Autodesk Fusion 360 part; units mm, degrees
(part 4 of 4)
  circle A338 centre (0, 0) radius 300
  spline S338 degree 3 poles (61.4407, -278.2986) (59.9759, -276.2105) (58.7077, -274.2475) (57.6132, -272.4294) knots 0 0 0 0 1 1 1 1
  spline S339 degree 3 poles (278.2308, -11.1655) (280.2066, -11.94) (282.3543, -12.8615) (284.6582, -13.9559) knots 0 0 0 0 1 1 1 1
  spline S340 degree 3 poles (276.3178, -10.4408) (276.936, -10.6668) (277.5738, -10.908) (278.2308, -11.1655) knots 0 0 0 0 1 1 1 1
  arc A339 (282.974, -33.9233) -> (283.4279, -29.8949) centre (0, 0) ccw
  spline S341 degree 3 poles (276.1699, -35.5976) (275.4792, -35.7415) (274.81, -35.8724) (274.1626, -35.9916) knots 0 0 0 0 1 1 1 1
  spline S342 degree 3 poles (275.2312, -42.2473) (277.1078, -43.2382) (279.1389, -44.3943) (281.3058, -45.7398) knots 0 0 0 0 1 1 1 1
  arc A340 (276.0555, -10.0506) -> (276.3178, -10.4408) centre (276.4552, -10.0652) ccw
  arc A341 (276.0555, -10.0506) -> (276.1847, -5.4437) centre (0, 0) ccw
  arc A342 (71.6656, -267.0666) -> (71.2268, -266.8977) centre (71.3299, -267.2842) ccw
  spline S343 degree 3 poles (280.6267, -49.7364) (278.137, -50.2907) (275.8381, -50.7111) (273.7395, -51.0266) knots 0 0 0 0 1 1 1 1
  arc A343 (280.6267, -49.7364) -> (281.3058, -45.7398) centre (0, 0) ccw
  arc A344 (273.1944, -40.8958) -> (273.4114, -41.313) centre (273.59, -40.9551) ccw
  spline S344 degree 3 poles (272.4294, -57.6132) (274.2475, -58.7077) (276.2105, -59.9759) (278.2986, -61.4407) knots 0 0 0 0 1 1 1 1
  spline S345 degree 3 poles (277.3965, -65.393) (274.8797, -65.8068) (272.5608, -66.0977) (270.4478, -66.295) knots 0 0 0 0 1 1 1 1
  arc A345 (257.2447, -100.662) -> (257.3634, -101.1169) centre (257.6171, -100.8077) ccw
  arc A346 (236.7485, -142.3298) -> (239.0901, -138.3603) centre (0, 0) ccw
  arc A347 (262.5234, -110.9347) -> (264.0748, -107.1894) centre (0, 0) ccw
  spline S346 degree 3 poles (252.7789, -116.7899) (254.3079, -118.2616) (255.9395, -119.9348) (257.6492, -121.8275) knots 0 0 0 0 1 1 1 1
  arc A348 (246.8902, -124.5221) -> (246.4719, -124.7367) centre (246.8288, -124.9173) ccw
  arc A349 (240.232, -153.3416) -> (242.3888, -149.9091) centre (0, 0) ccw
  arc A350 (244.3566, -128.8313) -> (244.4236, -129.2967) centre (244.7104, -129.0178) ccw
  arc A351 (236.7485, -142.3298) -> (236.7894, -142.7982) centre (237.0914, -142.5359) ccw
  spline S347 degree 3 poles (255.5218, -110.66) (254.8182, -110.607) (254.1389, -110.5476) (253.4839, -110.4829) knots 0 0 0 0 1 1 1 1
  arc A352 (248.452, -139.6305) -> (250.4129, -136.0824) centre (0, 0) ccw
  spline S348 degree 3 poles (248.9151, -124.8131) (248.2155, -124.7208) (247.5406, -124.6234) (246.8902, -124.5221) knots 0 0 0 0 1 1 1 1
  spline S349 degree 3 poles (248.452, -139.6305) (245.919, -139.3314) (243.6102, -138.969) (241.5251, -138.5736) knots 0 0 0 0 1 1 1 1
  arc A353 (262.4841, -86.0798) -> (263.8837, -81.6887) centre (0, 0) ccw
  arc A354 (262.4841, -86.0798) -> (262.6282, -86.5274) centre (262.8642, -86.2044) ccw
  spline S350 degree 3 poles (238.1131, -144.3578) (239.4677, -145.9914) (240.9017, -147.8368) (242.3888, -149.9091) knots 0 0 0 0 1 1 1 1
  spline S351 degree 3 poles (229.6443, -157.4818) (230.9052, -159.1888) (232.2335, -161.1117) (233.602, -163.2641) knots 0 0 0 0 1 1 1 1
  arc A355 (231.3958, -151.382) -> (230.9561, -151.5485) centre (231.2905, -151.7679) ccw
  spline S352 degree 3 poles (258.9296, -102.4328) (260.5388, -103.8164) (262.2616, -105.3955) (264.0748, -107.1894) knots 0 0 0 0 1 1 1 1
  spline S353 degree 3 poles (251.2888, -115.3883) (251.7735, -115.8336) (252.2705, -116.3006) (252.7789, -116.7899) knots 0 0 0 0 1 1 1 1
  arc A356 (257.2447, -100.662) -> (258.8882, -96.3563) centre (0, 0) ccw
  spline S354 degree 3 poles (266.3051, -81.3548) (265.6, -81.381) (264.9183, -81.398) (264.2602, -81.407) knots 0 0 0 0 1 1 1 1
  arc A357 (251.1958, -114.9274) -> (251.2888, -115.3883) centre (251.5595, -115.0938) ccw
  spline S355 degree 3 poles (262.6282, -86.5274) (263.1597, -86.9156) (263.7058, -87.324) (264.2658, -87.7533) knots 0 0 0 0 1 1 1 1
  arc A358 (259.2799, -96.0962) -> (258.8882, -96.3563) centre (259.2631, -96.4958) ccw
  spline S356 degree 3 poles (262.5234, -110.9347) (259.9728, -110.9211) (257.638, -110.8195) (255.5218, -110.66) knots 0 0 0 0 1 1 1 1
  arc A359 (244.3566, -128.8313) -> (246.4719, -124.7367) centre (0, 0) ccw
  arc A360 (255.8902, -125.48) -> (257.6492, -121.8275) centre (0, 0) ccw
  spline S357 degree 3 poles (255.8902, -125.48) (253.3445, -125.3234) (251.019, -125.091) (248.9151, -124.8131) knots 0 0 0 0 1 1 1 1
  spline S358 degree 3 poles (244.4236, -129.2967) (244.8826, -129.7685) (245.3526, -130.2625) (245.8327, -130.7796) knots 0 0 0 0 1 1 1 1
  spline S359 degree 3 poles (233.3753, -151.898) (232.6905, -151.7279) (232.0307, -151.5555) (231.3958, -151.382) knots 0 0 0 0 1 1 1 1
  spline S360 degree 3 poles (236.7894, -142.7982) (237.2212, -143.295) (237.6627, -143.8146) (238.1131, -144.3578) knots 0 0 0 0 1 1 1 1
  arc A361 (273.2935, -80.8439) -> (274.4157, -76.9484) centre (0, 0) ccw
  spline S361 degree 3 poles (240.232, -153.3416) (237.7197, -152.901) (235.4349, -152.4097) (233.3753, -151.898) knots 0 0 0 0 1 1 1 1
  arc A362 (264.2602, -81.407) -> (263.8837, -81.6887) centre (264.2658, -81.807) ccw
  spline S362 degree 3 poles (228.4101, -155.8505) (228.8134, -156.3707) (229.2251, -156.9142) (229.6443, -157.4818) knots 0 0 0 0 1 1 1 1
  arc A363 (228.3956, -155.3805) -> (228.4101, -155.8505) centre (228.7263, -155.6055) ccw
  spline S363 degree 3 poles (268.3306, -96.0404) (265.7832, -96.1698) (263.4464, -96.1992) (261.3246, -96.1587) knots 0 0 0 0 1 1 1 1
  arc A364 (231.2561, -166.5703) -> (233.602, -163.2641) centre (0, 0) ccw
  arc A365 (251.1958, -114.9274) -> (253.0782, -110.7207) centre (0, 0) ccw
  spline S364 degree 3 poles (241.5251, -138.5736) (240.8319, -138.4421) (240.1635, -138.307) (239.5198, -138.1694) knots 0 0 0 0 1 1 1 1
  spline S365 degree 3 poles (273.2935, -80.8439) (270.7574, -81.1159) (268.4259, -81.2764) (266.3051, -81.3548) knots 0 0 0 0 1 1 1 1
  spline S366 degree 3 poles (245.8327, -130.7796) (247.2768, -132.3347) (248.812, -134.0968) (250.4129, -136.0824) knots 0 0 0 0 1 1 1 1
  arc A366 (228.3956, -155.3805) -> (230.9561, -151.5485) centre (0, 0) ccw
  spline S367 degree 3 poles (261.3246, -96.1587) (260.6191, -96.1452) (259.9375, -96.124) (259.2799, -96.0962) knots 0 0 0 0 1 1 1 1
  spline S368 degree 3 poles (231.2561, -166.5703) (228.7725, -165.9895) (226.5188, -165.3708) (224.4912, -164.7445) knots 0 0 0 0 1 1 1 1
  spline S369 degree 3 poles (220.453, -170.1103) (221.6162, -171.8853) (222.8345, -173.8797) (224.0802, -176.1054) knots 0 0 0 0 1 1 1 1
  spline S370 degree 3 poles (224.4912, -164.7445) (223.817, -164.5362) (223.1679, -164.3272) (222.5437, -164.1184) knots 0 0 0 0 1 1 1 1
  arc A367 (219.324, -167.9423) -> (222.0953, -164.2599) centre (0, 0) ccw
  arc A368 (239.5198, -138.1694) -> (239.0901, -138.3603) centre (239.4363, -138.5606) ccw
  arc A369 (222.5437, -164.1184) -> (222.0953, -164.2599) centre (222.4169, -164.4977) ccw
  spline S371 degree 3 poles (219.3122, -168.4123) (219.6856, -168.9543) (220.0662, -169.5201) (220.453, -170.1103) knots 0 0 0 0 1 1 1 1
  spline S372 degree 3 poles (264.2658, -87.7533) (265.9499, -89.0445) (267.7586, -90.5246) (269.6695, -92.214) knots 0 0 0 0 1 1 1 1
  arc A370 (253.4839, -110.4829) -> (253.0782, -110.7207) centre (253.4447, -110.881) ccw
  arc A371 (268.3306, -96.0404) -> (269.6695, -92.214) centre (0, 0) ccw
  spline S373 degree 3 poles (257.3634, -101.1169) (257.8723, -101.5344) (258.3946, -101.9727) (258.9296, -102.4328) knots 0 0 0 0 1 1 1 1
  spline S374 degree 3 poles (200.0205, -193.7236) (200.9776, -195.6177) (201.965, -197.7359) (202.9537, -200.0871) knots 0 0 0 0 1 1 1 1
  spline S375 degree 3 poles (188.0034, -202.769) (188.2808, -203.3659) (188.5612, -203.9875) (188.8436, -204.6341) knots 0 0 0 0 1 1 1 1
  arc A372 (188.0938, -202.3076) -> (191.4428, -199.1414) centre (0, 0) ccw
  arc A373 (176.4544, -212.5358) -> (176.3383, -212.9914) centre (176.71, -212.8436) ccw
  arc A374 (212.9914, -176.3383) -> (212.5358, -176.4544) centre (212.8436, -176.71) ccw
  spline S376 degree 3 poles (200.0871, -202.9537) (197.7359, -201.965) (195.6177, -200.9776) (193.7236, -200.0205) knots 0 0 0 0 1 1 1 1
  spline S377 degree 3 poles (188.3926, -213.8534) (186.1006, -212.7344) (184.041, -211.6298) (182.2036, -210.568) knots 0 0 0 0 1 1 1 1
  spline S378 degree 3 poles (188.8436, -204.6341) (189.6931, -206.5789) (190.5602, -208.7491) (191.4154, -211.152) knots 0 0 0 0 1 1 1 1
  spline S379 degree 3 poles (177.0726, -214.9007) (177.8117, -216.89) (178.5557, -219.1055) (179.2749, -221.5526) knots 0 0 0 0 1 1 1 1
  spline S380 degree 3 poles (210.568, -182.2036) (211.6298, -184.041) (212.7344, -186.1006) (213.8534, -188.3926) knots 0 0 0 0 1 1 1 1
  arc A375 (155.8505, -228.4101) -> (155.3805, -228.3956) centre (155.6055, -228.7263) ccw
  spline S381 degree 3 poles (157.4818, -229.6443) (156.9142, -229.2251) (156.3707, -228.8134) (155.8505, -228.4101) knots 0 0 0 0 1 1 1 1
  arc A376 (199.1414, -191.4428) -> (202.3076, -188.0938) centre (0, 0) ccw
  arc A377 (149.9091, -242.3888) -> (153.3416, -240.232) centre (0, 0) ccw
  arc A378 (151.5485, -230.9561) -> (151.382, -231.3958) centre (151.7679, -231.2905) ccw
  spline S382 degree 3 poles (214.9007, -177.0726) (214.2393, -176.8269) (213.6029, -176.5818) (212.9914, -176.3383) knots 0 0 0 0 1 1 1 1
  arc A379 (200.0871, -202.9537) -> (202.9537, -200.0871) centre (0, 0) ccw
  spline S383 degree 3 poles (193.7236, -200.0205) (193.0938, -199.7023) (192.489, -199.3874) (191.9086, -199.077) knots 0 0 0 0 1 1 1 1
  arc A380 (151.5485, -230.9561) -> (155.3805, -228.3956) centre (0, 0) ccw
  arc A381 (202.769, -188.0034) -> (202.3076, -188.0938) centre (202.6005, -188.3662) ccw
  spline S384 degree 3 poles (211.152, -191.4154) (208.7491, -190.5602) (206.5789, -189.6931) (204.6341, -188.8436) knots 0 0 0 0 1 1 1 1
  spline S385 degree 3 poles (204.6341, -188.8436) (203.9875, -188.5612) (203.3659, -188.2808) (202.769, -188.0034) knots 0 0 0 0 1 1 1 1
  arc A382 (191.9086, -199.077) -> (191.4428, -199.1414) centre (191.72, -199.4298) ccw
  arc A383 (219.324, -167.9423) -> (219.3122, -168.4123) centre (219.6416, -168.1855) ccw
  spline S386 degree 3 poles (176.1054, -224.0802) (173.8797, -222.8345) (171.8853, -221.6162) (170.1103, -220.453) knots 0 0 0 0 1 1 1 1
  arc A384 (176.1054, -224.0802) -> (179.2749, -221.5526) centre (0, 0) ccw
  arc A385 (163.2641, -233.602) -> (166.5703, -231.2561) centre (0, 0) ccw
  spline S387 degree 3 poles (164.7445, -224.4912) (165.3708, -226.5188) (165.9895, -228.7725) (166.5703, -231.2561) knots 0 0 0 0 1 1 1 1
  arc A386 (168.4123, -219.3122) -> (167.9423, -219.324) centre (168.1855, -219.6416) ccw
  arc A387 (188.0938, -202.3076) -> (188.0034, -202.769) centre (188.3662, -202.6005) ccw
  arc A388 (211.152, -191.4154) -> (213.8534, -188.3926) centre (0, 0) ccw
  spline S388 degree 3 poles (182.2036, -210.568) (181.5927, -210.2149) (181.0064, -209.8667) (180.4443, -209.5242) knots 0 0 0 0 1 1 1 1
  arc A389 (209.5624, -179.9757) -> (209.5242, -180.4443) centre (209.8658, -180.2363) ccw
  arc A390 (176.4544, -212.5358) -> (179.9757, -209.5624) centre (0, 0) ccw
  spline S389 degree 3 poles (199.077, -191.9086) (199.3874, -192.489) (199.7023, -193.0938) (200.0205, -193.7236) knots 0 0 0 0 1 1 1 1
  arc A391 (180.4443, -209.5242) -> (179.9757, -209.5624) centre (180.2363, -209.8658) ccw
  arc A392 (164.2599, -222.0953) -> (164.1184, -222.5437) centre (164.4977, -222.4169) ccw
  spline S390 degree 3 poles (164.1184, -222.5437) (164.3272, -223.1679) (164.5362, -223.817) (164.7445, -224.4912) knots 0 0 0 0 1 1 1 1
  arc A393 (209.5624, -179.9757) -> (212.5358, -176.4544) centre (0, 0) ccw
  spline S391 degree 3 poles (170.1103, -220.453) (169.5201, -220.0662) (168.9543, -219.6856) (168.4123, -219.3122) knots 0 0 0 0 1 1 1 1
  arc A394 (164.2599, -222.0953) -> (167.9423, -219.324) centre (0, 0) ccw
  spline S392 degree 3 poles (163.2641, -233.602) (161.1117, -232.2335) (159.1888, -230.9052) (157.4818, -229.6443) knots 0 0 0 0 1 1 1 1
  spline S393 degree 3 poles (151.898, -233.3753) (152.4097, -235.4349) (152.901, -237.7197) (153.3416, -240.232) knots 0 0 0 0 1 1 1 1
  arc A395 (188.3926, -213.8534) -> (191.4154, -211.152) centre (0, 0) ccw
  spline S394 degree 3 poles (151.382, -231.3958) (151.5555, -232.0307) (151.7279, -232.6905) (151.898, -233.3753) knots 0 0 0 0 1 1 1 1
  spline S395 degree 3 poles (176.3383, -212.9914) (176.5818, -213.6029) (176.8269, -214.2393) (177.0726, -214.9007) knots 0 0 0 0 1 1 1 1
  arc A396 (221.5526, -179.2749) -> (224.0802, -176.1054) centre (0, 0) ccw
  spline S396 degree 3 poles (209.5242, -180.4443) (209.8667, -181.0064) (210.2149, -181.5927) (210.568, -182.2036) knots 0 0 0 0 1 1 1 1
  spline S397 degree 3 poles (221.5526, -179.2749) (219.1055, -178.5557) (216.89, -177.8117) (214.9007, -177.0726) knots 0 0 0 0 1 1 1 1
  arc A397 (199.1414, -191.4428) -> (199.077, -191.9086) centre (199.4298, -191.72) ccw
  spline S398 degree 3 poles (166.5703, 231.2561) (165.9895, 228.7725) (165.3708, 226.5188) (164.7445, 224.4912) knots 0 0 0 0 1 1 1 1
  arc A398 (167.9423, 219.324) -> (164.2599, 222.0953) centre (0, 0) ccw
  spline S399 degree 3 poles (277.167, 26.7485) (276.5255, 26.4545) (275.9023, 26.1779) (275.2977, 25.9177) knots 0 0 0 0 1 1 1 1
  spline S400 degree 3 poles (155.8505, 228.4101) (156.3707, 228.8134) (156.9142, 229.2251) (157.4818, 229.6443) knots 0 0 0 0 1 1 1 1
  arc A399 (138.1694, 239.5198) -> (138.3603, 239.0901) centre (138.5606, 239.4363) ccw
  spline S401 degree 3 poles (168.4123, 219.3122) (168.9543, 219.6856) (169.5201, 220.0662) (170.1103, 220.453) knots 0 0 0 0 1 1 1 1
  spline S402 degree 3 poles (179.2749, 221.5526) (178.5557, 219.1055) (177.8117, 216.89) (177.0726, 214.9007) knots 0 0 0 0 1 1 1 1
  spline S403 degree 3 poles (276.1699, 35.5976) (278.2476, 35.165) (280.5193, 34.6163) (282.974, 33.9233) knots 0 0 0 0 1 1 1 1
  arc A400 (276.1847, 5.4437) -> (276.4685, 5.0688) centre (276.5847, 5.4516) ccw
  arc A401 (166.5703, 231.2561) -> (163.2641, 233.602) centre (0, 0) ccw
  spline S404 degree 3 poles (275.2312, 42.2473) (274.6072, 41.9178) (274.0004, 41.6067) (273.4114, 41.313) knots 0 0 0 0 1 1 1 1
  spline S405 degree 3 poles (170.1103, 220.453) (171.8853, 221.6162) (173.8797, 222.8345) (176.1054, 224.0802) knots 0 0 0 0 1 1 1 1
  arc A402 (275.2977, 25.9177) -> (275.0576, 25.5134) centre (275.4559, 25.5503) ccw
  spline S406 degree 3 poles (180.4443, 209.5242) (181.0064, 209.8667) (181.5927, 210.2149) (182.2036, 210.568) knots 0 0 0 0 1 1 1 1
  spline S407 degree 3 poles (139.6305, 248.452) (139.3314, 245.919) (138.969, 243.6102) (138.5736, 241.5251) knots 0 0 0 0 1 1 1 1
  arc A403 (179.9757, 209.5624) -> (176.4544, 212.5358) centre (0, 0) ccw
  spline S408 degree 3 poles (283.4279, 29.8949) (281.1889, 28.673) (279.0963, 27.6326) (277.167, 26.7485) knots 0 0 0 0 1 1 1 1
  arc A404 (275.445, 20.921) -> (275.0576, 25.5134) centre (0, 0) ccw
  spline S409 degree 3 poles (284.6582, 13.9559) (282.3543, 12.8615) (280.2066, 11.94) (278.2308, 11.1655) knots 0 0 0 0 1 1 1 1
  spline S410 degree 3 poles (144.3578, 238.1131) (145.9914, 239.4677) (147.8368, 240.9017) (149.9091, 242.3888) knots 0 0 0 0 1 1 1 1
  arc A405 (283.4279, 29.8949) -> (282.974, 33.9233) centre (0, 0) ccw
  arc A406 (155.3805, 228.3956) -> (155.8505, 228.4101) centre (155.6055, 228.7263) ccw
  spline S411 degree 3 poles (275.7494, 20.5626) (276.389, 20.4073) (277.0498, 20.239) (277.7315, 20.0566) knots 0 0 0 0 1 1 1 1
  spline S412 degree 3 poles (278.2308, 11.1655) (277.5738, 10.908) (276.936, 10.6668) (276.3178, 10.4408) knots 0 0 0 0 1 1 1 1
  arc A407 (273.8386, 36.3324) -> (273.1944, 40.8958) centre (0, 0) ccw
  spline S413 degree 3 poles (138.5736, 241.5251) (138.4421, 240.8319) (138.307, 240.1635) (138.1694, 239.5198) knots 0 0 0 0 1 1 1 1
  arc A408 (155.3805, 228.3956) -> (151.5485, 230.9561) centre (0, 0) ccw
  arc A409 (151.382, 231.3958) -> (151.5485, 230.9561) centre (151.7679, 231.2905) ccw
  arc A410 (179.9757, 209.5624) -> (180.4443, 209.5242) centre (180.2363, 209.8658) ccw
  arc A411 (281.3058, 45.7398) -> (280.6267, 49.7364) centre (0, 0) ccw
  spline S414 degree 3 poles (281.3058, 45.7398) (279.1389, 44.3943) (277.1078, 43.2382) (275.2312, 42.2473) knots 0 0 0 0 1 1 1 1
  arc A412 (179.2749, 221.5526) -> (176.1054, 224.0802) centre (0, 0) ccw
  arc A413 (176.3383, 212.9914) -> (176.4544, 212.5358) centre (176.71, 212.8436) ccw
  spline S415 degree 3 poles (177.0726, 214.9007) (176.8269, 214.2393) (176.5818, 213.6029) (176.3383, 212.9914) knots 0 0 0 0 1 1 1 1
  arc A414 (191.4154, 211.152) -> (188.3926, 213.8534) centre (0, 0) ccw
  arc A415 (273.8386, 36.3324) -> (274.1626, 35.9916) centre (274.2352, 36.385) ccw
  spline S416 degree 3 poles (277.7315, 20.0566) (279.7816, 19.5082) (282.0189, 18.833) (284.4309, 18.0035) knots 0 0 0 0 1 1 1 1
  arc A416 (276.1847, 5.4437) -> (276.0555, 10.0506) centre (0, 0) ccw
  spline S417 degree 3 poles (153.3416, 240.232) (152.901, 237.7197) (152.4097, 235.4349) (151.898, 233.3753) knots 0 0 0 0 1 1 1 1
  spline S418 degree 3 poles (151.898, 233.3753) (151.7279, 232.6905) (151.5555, 232.0307) (151.382, 231.3958) knots 0 0 0 0 1 1 1 1
  arc A417 (273.4114, 41.313) -> (273.1944, 40.8958) centre (273.59, 40.9551) ccw
  arc A418 (164.1184, 222.5437) -> (164.2599, 222.0953) centre (164.4977, 222.4169) ccw
  arc A419 (167.9423, 219.324) -> (168.4123, 219.3122) centre (168.1855, 219.6416) ccw
  spline S419 degree 3 poles (164.7445, 224.4912) (164.5362, 223.817) (164.3272, 223.1679) (164.1184, 222.5437) knots 0 0 0 0 1 1 1 1
  spline S420 degree 3 poles (273.7395, 51.0266) (275.8381, 50.7111) (278.137, 50.2907) (280.6267, 49.7364) knots 0 0 0 0 1 1 1 1
  arc A420 (284.6582, 13.9559) -> (284.4309, 18.0035) centre (0, 0) ccw
  arc A421 (142.3298, 236.7485) -> (142.7982, 236.7894) centre (142.5359, 237.0914) ccw
  spline S421 degree 3 poles (142.7982, 236.7894) (143.295, 237.2212) (143.8146, 237.6627) (144.3578, 238.1131) knots 0 0 0 0 1 1 1 1
  arc A422 (153.3416, 240.232) -> (149.9091, 242.3888) centre (0, 0) ccw
  spline S422 degree 3 poles (274.1626, 35.9916) (274.81, 35.8724) (275.4792, 35.7415) (276.1699, 35.5976) knots 0 0 0 0 1 1 1 1
  arc A423 (275.445, 20.921) -> (275.7494, 20.5626) centre (275.8439, 20.9513) ccw
  arc A424 (276.3178, 10.4408) -> (276.0555, 10.0506) centre (276.4552, 10.0652) ccw
  arc A425 (142.3298, 236.7485) -> (138.3603, 239.0901) centre (0, 0) ccw
  spline S423 degree 3 poles (157.4818, 229.6443) (159.1888, 230.9052) (161.1117, 232.2335) (163.2641, 233.602) knots 0 0 0 0 1 1 1 1
  arc A426 (213.8534, 188.3926) -> (211.152, 191.4154) centre (0, 0) ccw
  arc A427 (202.3076, 188.0938) -> (202.769, 188.0034) centre (202.6005, 188.3662) ccw
  spline S424 degree 3 poles (202.9537, 200.0871) (201.965, 197.7359) (200.9776, 195.6177) (200.0205, 193.7236) knots 0 0 0 0 1 1 1 1
  spline S425 degree 3 poles (188.8436, 204.6341) (188.5612, 203.9875) (188.2808, 203.3659) (188.0034, 202.769) knots 0 0 0 0 1 1 1 1
  spline S426 degree 3 poles (204.6341, 188.8436) (206.5789, 189.6931) (208.7491, 190.5602) (211.152, 191.4154) knots 0 0 0 0 1 1 1 1
  arc A428 (224.0802, 176.1054) -> (221.5526, 179.2749) centre (0, 0) ccw
  arc A429 (212.5358, 176.4544) -> (209.5624, 179.9757) centre (0, 0) ccw
  arc A430 (191.4428, 199.1414) -> (191.9086, 199.077) centre (191.72, 199.4298) ccw
  spline S427 degree 3 poles (224.0802, 176.1054) (222.8345, 173.8797) (221.6162, 171.8853) (220.453, 170.1103) knots 0 0 0 0 1 1 1 1
  spline S428 degree 3 poles (224.4912, 164.7445) (226.5188, 165.3708) (228.7725, 165.9895) (231.2561, 166.5703) knots 0 0 0 0 1 1 1 1
  spline S429 degree 3 poles (233.602, 163.2641) (232.2335, 161.1117) (230.9052, 159.1888) (229.6443, 157.4818) knots 0 0 0 0 1 1 1 1
  spline S430 degree 3 poles (229.6443, 157.4818) (229.2251, 156.9142) (228.8134, 156.3707) (228.4101, 155.8505) knots 0 0 0 0 1 1 1 1
  arc A431 (230.9561, 151.5485) -> (231.3958, 151.382) centre (231.2905, 151.7679) ccw
  spline S431 degree 3 poles (233.3753, 151.898) (235.4349, 152.4097) (237.7197, 152.901) (240.232, 153.3416) knots 0 0 0 0 1 1 1 1
  spline S432 degree 3 poles (231.3958, 151.382) (232.0307, 151.5555) (232.6905, 151.7279) (233.3753, 151.898) knots 0 0 0 0 1 1 1 1
  arc A432 (222.0953, 164.2599) -> (219.324, 167.9423) centre (0, 0) ccw
  arc A433 (202.9537, 200.0871) -> (200.0871, 202.9537) centre (0, 0) ccw
  spline S433 degree 3 poles (213.8534, 188.3926) (212.7344, 186.1006) (211.6298, 184.041) (210.568, 182.2036) knots 0 0 0 0 1 1 1 1
  spline S434 degree 3 poles (212.9914, 176.3383) (213.6029, 176.5818) (214.2393, 176.8269) (214.9007, 177.0726) knots 0 0 0 0 1 1 1 1
  spline S435 degree 3 poles (222.5437, 164.1184) (223.1679, 164.3272) (223.817, 164.5362) (224.4912, 164.7445) knots 0 0 0 0 1 1 1 1
  arc A434 (233.602, 163.2641) -> (231.2561, 166.5703) centre (0, 0) ccw
  arc A435 (242.3888, 149.9091) -> (240.232, 153.3416) centre (0, 0) ccw
  arc A436 (188.0034, 202.769) -> (188.0938, 202.3076) centre (188.3662, 202.6005) ccw
  arc A437 (230.9561, 151.5485) -> (228.3956, 155.3805) centre (0, 0) ccw
  spline S436 degree 3 poles (191.9086, 199.077) (192.489, 199.3874) (193.0938, 199.7023) (193.7236, 200.0205) knots 0 0 0 0 1 1 1 1
  spline S437 degree 3 poles (193.7236, 200.0205) (195.6177, 200.9776) (197.7359, 201.965) (200.0871, 202.9537) knots 0 0 0 0 1 1 1 1
  spline S438 degree 3 poles (210.568, 182.2036) (210.2149, 181.5927) (209.8667, 181.0064) (209.5242, 180.4443) knots 0 0 0 0 1 1 1 1
  arc A438 (239.0901, 138.3603) -> (236.7485, 142.3298) centre (0, 0) ccw
  spline S439 degree 3 poles (238.1131, 144.3578) (237.6627, 143.8146) (237.2212, 143.295) (236.7894, 142.7982) knots 0 0 0 0 1 1 1 1
  arc A439 (236.7894, 142.7982) -> (236.7485, 142.3298) centre (237.0914, 142.5359) ccw
  arc A440 (239.0901, 138.3603) -> (239.5198, 138.1694) centre (239.4363, 138.5606) ccw
  spline S440 degree 3 poles (242.3888, 149.9091) (240.9017, 147.8368) (239.4677, 145.9914) (238.1131, 144.3578) knots 0 0 0 0 1 1 1 1
  spline S441 degree 3 poles (239.5198, 138.1694) (240.1635, 138.307) (240.8319, 138.4421) (241.5251, 138.5736) knots 0 0 0 0 1 1 1 1
  spline S442 degree 3 poles (200.0205, 193.7236) (199.7023, 193.0938) (199.3874, 192.489) (199.077, 191.9086) knots 0 0 0 0 1 1 1 1
  spline S443 degree 3 poles (182.2036, 210.568) (184.041, 211.6298) (186.1006, 212.7344) (188.3926, 213.8534) knots 0 0 0 0 1 1 1 1
  arc A441 (202.3076, 188.0938) -> (199.1414, 191.4428) centre (0, 0) ccw
  spline S444 degree 3 poles (191.4154, 211.152) (190.5602, 208.7491) (189.6931, 206.5789) (188.8436, 204.6341) knots 0 0 0 0 1 1 1 1
  arc A442 (219.3122, 168.4123) -> (219.324, 167.9423) centre (219.6416, 168.1855) ccw
  arc A443 (228.4101, 155.8505) -> (228.3956, 155.3805) centre (228.7263, 155.6055) ccw
  spline S445 degree 3 poles (202.769, 188.0034) (203.3659, 188.2808) (203.9875, 188.5612) (204.6341, 188.8436) knots 0 0 0 0 1 1 1 1
  arc A444 (209.5242, 180.4443) -> (209.5624, 179.9757) centre (209.8658, 180.2363) ccw
  spline S446 degree 3 poles (214.9007, 177.0726) (216.89, 177.8117) (219.1055, 178.5557) (221.5526, 179.2749) knots 0 0 0 0 1 1 1 1
  arc A445 (222.0953, 164.2599) -> (222.5437, 164.1184) centre (222.4169, 164.4977) ccw
  arc A446 (199.077, 191.9086) -> (199.1414, 191.4428) centre (199.4298, 191.72) ccw
  arc A447 (191.4428, 199.1414) -> (188.0938, 202.3076) centre (0, 0) ccw
  arc A448 (212.5358, 176.4544) -> (212.9914, 176.3383) centre (212.8436, 176.71) ccw
  spline S447 degree 3 poles (220.453, 170.1103) (220.0662, 169.5201) (219.6856, 168.9543) (219.3122, 168.4123) knots 0 0 0 0 1 1 1 1
extrude "Extrude1''" add sketch "sketch 19514" along normal blind 8 separate body makes body 3 in component "Internal Gear (112 teeth)"
sketch "Sketch1 (3)" plane through (0, 0, 0) normal (0, 1, 0) x (1, 0, 0) in component "Internal Gear (112 teeth)"
  circle A0 centre (0, 0) radius 280 construction
component "Spur Gear (56 teeth)" placed x (1, 0, 0) y (0, 1, 0) z (0, 0, 1) at (0, 0, 0)
component "Spur Gear (28 teeth)" placed x (1, 0, 0) y (0, 1, 0) z (0, 0, 1) at (0, 0, 0)
component "Internal Gear (112 teeth)" placed x (1, 0, 0) y (0, 1, 0) z (0, 0, 1) at (0, 0, 0)
